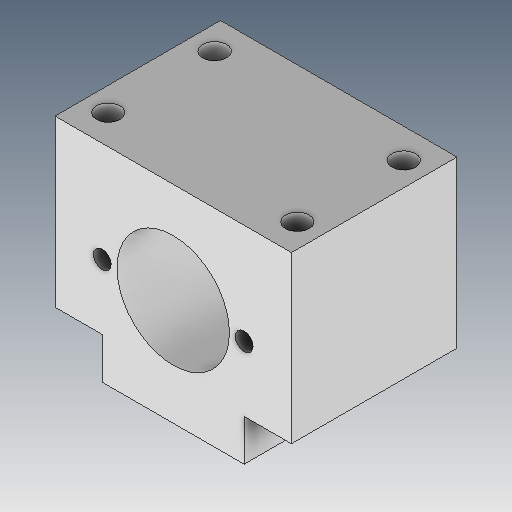
# Autodesk Inventor part: Soporte de Buje
Saved by Autodesk Inventor 2020 (Build 240168000, 168)
## iProperties
Created: 2020-05-08
Part Number: Soporte de Buje
Material: Aluminum 6061
Document SubType Name: Modeling
Designer: Pipi
Density: 2.7 g/cm^3
Appearance: Default
Mass: 57.6965 g
Surface Area: 82.5584 cm^2
Volume: 21.3691 cm^3
Author: Pipi
Autodesk Inventor part; units mm, degrees
ref_plane "YZ Plane" through (0, 0, 0) normal (1, 0, 0) x (0, 1, 0)
ref_plane "XZ Plane" through (0, 0, 0) normal (0, 1, 0) x (-1, 0, 0)
ref_plane "XY Plane" through (0, 0, 0) normal (0, 0, 1) x (1, 0, 0)
sketch "Boceto1" plane through (0, 0, 0) normal (0, 1, 0) x (-1, 0, 0)
  line L0 (40, 11) -> (40, 29.5)
  line L1 (40, 29.5) -> (0, 29.5)
  line L2 (0, 29.5) -> (0, 7.5)
  circle A0 centre (20, 12.5) radius 9.5
  line L3 (40, 11) -> (40, 1.5)
  line L4 (40, 1.5) -> (32, 1.5)
  line L5 (0, 7.5) -> (0, 1.5)
  line L6 (0, 1.5) -> (8, 1.5)
  line L7 (32, 1.5) -> (32, -5.5)
  line L8 (32, -5.5) -> (8, -5.5)
  line L9 (8, -5.5) -> (8, 1.5)
  point P0 (0, 0)
  point P1 (0, 0)
  dimension "d1" = 19
  dimension "d14" = 40
  dimension "d18" = 8
  dimension "d19" = 8
  dimension "d20" = 28
  dimension "d21" = 35
  dimension "d35" = 17
  dimension "d68" = 28
  constraints: 20 end point, 6 perpendicular, 3 vertical, 1 centre point
  measures "d1" diameter of A0
  measures "d14" distance of L0.end L1.end
  measures "d18" distance of L3.end L4.end
  measures "d19" distance of L5.end L6.end
  measures "d20" distance between parallel lines of L1 L4
  measures "d21" distance between parallel lines of L8 L1
  measures "d35" distance from line of L1 A0.centre
  measures "d68" distance between parallel lines of L1 L6
extrude "Extrusión1" add sketch "Boceto1" along normal blind 28
sketch "Boceto7" plane through (0, 0, 1.5) normal (0, 0, -1) x (-1, 0, 0)
  line L0 (0, 0) -> (0, 28) projected
  line L1 (0, 0) -> (4, 0)
  line L2 (40, 0) -> (0, 0) projected
  line L3 (4, 0) -> (4, 28)
  line L4 (40, 28) -> (0, 28) projected
  line L5 (4, 14) -> (4, 5)
  circle A0 centre (4, 5) radius 2
  circle A1 centre (4, 23) radius 2
  line L6 (40, 0) -> (40, 28) projected
  line L7 (40, 0) -> (36, 0)
  line L8 (36, 0) -> (36, 28)
  circle A2 centre (36, 5) radius 2
  circle A3 centre (36, 23) radius 2
  dimension "d24" = 4
  dimension "d25" = 4
  dimension "d26" = 5
  dimension "d27" = 5
  dimension "d28" = 4
  dimension "d29" = 4
  dimension "d30" = 4
  dimension "d31" = 5
  dimension "d32" = 5
  dimension "d60" = 4
  constraints: 10 end point, 9 point on line, 4 centre point, 2 perpendicular, 1 midpoint
  measures "d24" diameter of A0
  measures "d25" diameter of A1
  measures "d26" distance of L1.end A0.centre
  measures "d27" distance of L3.end A1.centre
  measures "d28" distance of L2.start L7.end
  measures "d29" diameter of A2
  measures "d30" diameter of A3
  measures "d31" distance of L7.end A2.centre
  measures "d32" distance of L8.end A3.centre
  measures "d60" distance between parallel lines of L0 L3
extrude "Extrusión4" cut sketch "Boceto7" against normal blind 28 contours A0 L3 | L3 A0 | A1 L3 | L3 A1 | A2 L8 | L8 A2 | A3 L8 | L8 A3
sketch "Boceto9" plane through (0, 28, 0) normal (0, 1, 0) x (1, 0, 0)
  circle A0 centre (-20, -12.5) radius 9.5 projected
  circle A1 centre (-8, -12.5) radius 1.5
  circle A2 centre (-32, -12.5) radius 1.5
  point P0 (0, 0)
  dimension "d36" = 12
  dimension "d38" = 3
  dimension "d39" = 3
  dimension "d61" = 12
  constraints: 2 centre point, 2 coincident
  measures "d36" distance of A0.centre point (-32, -12.5)
  measures "d38" diameter of A1
  measures "d39" diameter of A2
  measures "d61" distance of point (-8, -12.5) A0.centre
sketch "Boceto10" plane through (0, 0, 0) normal (0, -1, 0) x (1, 0, 0)
  circle A0 centre (-20, 12.5) radius 9.5 projected
  line L0 (-20, 12.5) -> (-8, 12.5)
  line L1 (-8, 12.5) -> (-32, 12.5)
  circle A1 centre (-32, 12.5) radius 1.5
  circle A2 centre (-8, 12.5) radius 1.5
  point P0 (0, 0)
  dimension "d40" = 12
  dimension "d41" = 24
  dimension "d42" = 3
  dimension "d43" = 3
  constraints: 4 end point, 2 centre point, 2 coincident, 1 horizontal, 1 point on line
  measures "d40" distance of L0.start L0.end
  measures "d41" distance of L0.end L1.end
  measures "d42" diameter of A1
  measures "d43" diameter of A2
hole "Agujero1" at (-32, 0, 12.5) at (-8, 0, 12.5) direction (0, 1, 0) diameter 3 depth 12.5 tip angle 118
hole "Agujero2" at (-8, 28, 12.5) at (-32, 28, 12.5) direction (0, -1, 0) diameter 3 depth 12.5 tip angle 118
thread "Rosca1" size "M3x0.5" class "6H" standard "ISO Metric profile" length 10
thread "Rosca2" size "M3x0.5" class "6H" standard "ISO Metric profile" length 10
thread "Rosca3" size "M3x0.5" class "6H" standard "ISO Metric profile" length 10
thread "Rosca4" size "M3x0.5" class "6H" standard "ISO Metric profile" length 10
equation "\"d68\" = d20"
